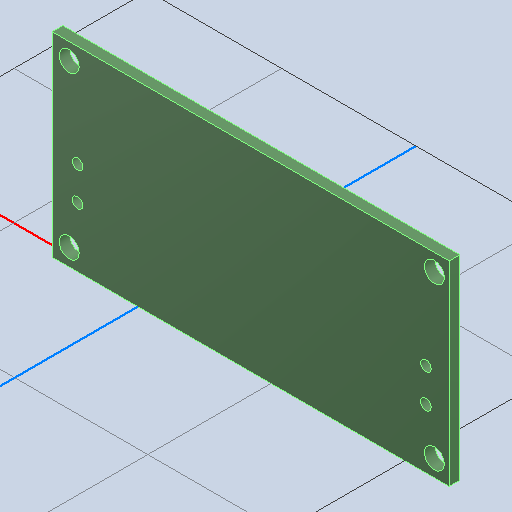
# Autodesk Inventor part: untitled.brdКонтур
Saved by Autodesk Inventor 2022 (Build 260153000, 153)
## iProperties
Created: 2022-02-26
Part Number: untitled.brdКонтур
Material: Типовые
Document SubType Name: Modeling
Designer: Petrov Ivan
Density: 1 g/cm^3
Appearance: Контур панели
Author: Petrov Ivan
Autodesk Inventor part; units mm, degrees
ref_plane "YZ Plane" through (0, 0, 0) normal (1, 0, 0) x (0, 1, 0)
ref_plane "XZ Plane" through (0, 0, 0) normal (0, 1, 0) x (-1, 0, 0)
ref_plane "XY Plane" through (0, 0, 0) normal (0, 0, 1) x (1, 0, 0)
sketch "Эскиз1" plane through (0, 0, 0) normal (0, 0, 1) x (1, 0, 0)
  line L0 (-12.7, 0) -> (46.66, 0)
  line L1 (46.66, 0) -> (46.66, 29.2)
  line L2 (46.66, 29.2) -> (-12.7, 29.2)
  line L3 (-12.7, 29.2) -> (-12.7, 0)
  circle A0 centre (-8.89, 13.97) radius 0.8
  circle A1 centre (-8.89, 8.97) radius 0.8
  circle A2 centre (43.18, 8.89) radius 0.8
  circle A3 centre (43.18, 13.89) radius 0.8
  circle A4 centre (-10.16, 26.67) radius 1.5
  circle A5 centre (44.45, 26.67) radius 1.5
  circle A6 centre (44.45, 2.54) radius 1.5
  circle A7 centre (-10.16, 2.54) radius 1.5
  constraints: 8 centre point, 8 end point
extrude "untitled.brdКонтур" add sketch "Эскиз1" along normal blind 1.6
